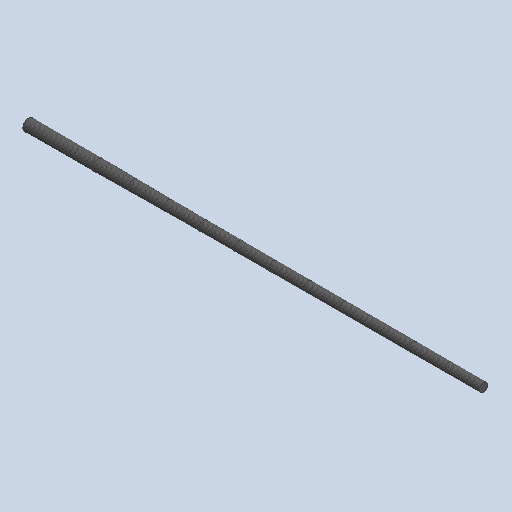
# Autodesk Inventor part: 1P.02.01.02-RN-MainSpar
Saved by Autodesk Inventor 2025.2 (Build 292293000, 293)
## iProperties
Created: 2025-01-16
Part Number: 1P.02.01.02-RN-MainSpar
Material: CFRP
Document SubType Name: Modeling
Designer: hjbre
Density: 1.43 g/cm^3
Appearance: Carbon Fiber
Author: hjbre
Autodesk Inventor part; units mm, degrees
ref_plane "YZ Plane" through (0, 0, 0) normal (1, 0, 0) x (0, 1, 0)
ref_plane "XZ Plane" through (0, 0, 0) normal (0, 1, 0) x (-1, 0, 0)
ref_plane "XY Plane" through (0, 0, 0) normal (0, 0, 1) x (1, 0, 0)
sketch "Sketch1" plane through (0, 0, 0) normal (0, 0, 1) x (1, 0, 0)
  line L0 (-100, 0) -> (1200, 0)
  line L1 (-100, 0) -> (-100, 16.7)
  line L2 (100, 0) -> (100, 16.15)
  line L3 (200, 0) -> (200, 15.15)
  line L4 (300, 0) -> (300, 14.2)
  line L5 (400, 0) -> (400, 13.69)
  line L6 (500, 0) -> (500, 13.5)
  line L7 (600, 0) -> (600, 13.29)
  line L8 (700, 0) -> (700, 13.175)
  line L9 (800, 0) -> (800, 12.95)
  line L10 (900, 0) -> (900, 12.9)
  line L11 (1000, 0) -> (1000, 12.85)
  line L12 (1100, 0) -> (1100, 12.4)
  line L13 (1200, 0) -> (1200, 12.4)
  line L14 (1200, 0) -> (1200, 11.25)
  line L15 (-100, 16.7) -> (100, 16.15)
  line L16 (100, 16.15) -> (200, 15.15)
  line L17 (200, 15.15) -> (300, 14.2)
  line L18 (300, 14.2) -> (400, 13.69)
  line L19 (400, 13.69) -> (500, 13.5)
  line L20 (500, 13.5) -> (600, 13.29)
  line L21 (600, 13.29) -> (700, 13.175)
  line L22 (700, 13.175) -> (800, 12.95)
  line L23 (800, 12.95) -> (900, 12.9)
  line L24 (900, 12.9) -> (1000, 12.85)
  line L25 (1000, 12.85) -> (1100, 12.4)
  line L26 (1100, 12.4) -> (1200, 12.4)
  line L27 (1200, 12.4) -> (1200, 11.25)
  point P0 (0, 0)
  point P1 (1100, 12.3857)
  point P2 (1090, 12.3713)
  point P3 (1080, 12.357)
  point P4 (1070, 12.3426)
  point P5 (1060, 12.3283)
  point P6 (1050, 12.3139)
  point P7 (1010, 11.54)
  point P8 (1020, 11.7067)
  point P9 (1030, 12.2852)
  point P10 (1040, 12.2996)
  dimension "d0" = 1300
  dimension "d1" = 100
  dimension "d2" = 100
  dimension "d3" = 100
  dimension "d4" = 100
  dimension "d5" = 100
  dimension "d6" = 100
  dimension "d7" = 100
  dimension "d8" = 100
  dimension "d9" = 100
  dimension "d10" = 100
  dimension "d11" = 100
  dimension "d12" = 100
  dimension "d13" = 16.7
  dimension "d14" = 16.15
  dimension "d15" = 15.15
  dimension "d16" = 14.2
  dimension "d17" = 13.69
  dimension "d18" = 13.5
  dimension "d19" = 13.29
  dimension "d20" = 13.175
  dimension "d21" = 12.95
  dimension "d22" = 12.9
  dimension "d23" = 12.85
  dimension "d24" = 12.4
  dimension "d25" = 12.4
  dimension "d26" = 11.25
  dimension "d31" = 100
  constraints: 54 end point, 14 vertical, 15 other
  measures "d0" distance of L1.start L14.start
  measures "d1" distance of L2.start point (0, 0)
  measures "d2" distance of L3.start L2.start
  measures "d3" distance of L4.start L3.start
  measures "d4" distance of L5.start L4.start
  measures "d5" distance of L6.start L5.start
  measures "d6" distance of L7.start L6.start
  measures "d7" distance of L8.start L7.start
  measures "d8" distance of L9.start L8.start
  measures "d9" distance of L10.start L9.start
  measures "d10" distance of L11.start L10.start
  measures "d11" distance of L12.start L11.start
  measures "d12" distance of L13.start L12.start
  measures "d13" distance of L1.start L1.end
  measures "d14" distance of L2.start L2.end
  measures "d15" distance of L3.start L3.end
  measures "d16" distance of L4.start L4.end
  measures "d17" distance of L5.start L5.end
  measures "d18" distance of L6.start L6.end
  measures "d19" distance of L7.start L7.end
  measures "d20" distance of L8.start L8.end
  measures "d21" distance of L9.start L9.end
  measures "d22" distance of L10.start L10.end
  measures "d23" distance of L11.start L11.end
  measures "d24" distance of L12.start L12.end
  measures "d25" distance of L13.start L13.end
  measures "d26" distance of L14.start L14.end
  measures "d31" horizontal distance of point (0, 0) L1.end
revolve "Revolution4" add sketch "Sketch1" angle 360 about axis through (-100, 0, 0) along (1, 0, 0)
body "Solid2"
